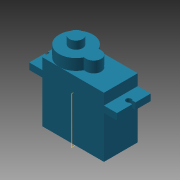
# Autodesk Inventor part: Servo
Saved by Autodesk Inventor 2014 SP1 (Build 180222100, 222)
## iProperties
Created: 2017-01-16
Part Number: Servo
Material: Generic
Document SubType Name: Modeling
Designer: danielsikar
Density: 1 g/cm^3
Appearance: Turquoise
Author: danielsikar
Autodesk Inventor part; units mm, degrees
ref_plane "YZ Plane" through (0, 0, 0) normal (1, 0, 0) x (0, 1, 0)
ref_plane "XZ Plane" through (0, 0, 0) normal (0, 1, 0) x (-1, 0, 0)
ref_plane "XY Plane" through (0, 0, 0) normal (0, 0, 1) x (1, 0, 0)
sketch "Sketch1" plane through (0, 0, 0) normal (0, 0, 1) x (1, 0, 0)
  line L0 (0, 0) -> (22.8, 0)
  line L1 (22.8, 0) -> (22.8, 12.5)
  line L2 (22.8, 12.5) -> (0, 12.5)
  line L3 (0, 12.5) -> (0, 0)
  dimension "d0" = 22.8
  dimension "d1" = 12.5
  constraints: 8 end point, 2 parallel, 1 horizontal, 1 perpendicular
  measures "d0" distance of L2.end L1.end
  measures "d1" distance of L1.end L0.end
extrude "Extrusion1" add sketch "Sketch1" along normal blind 22.1
sketch "Sketch2" plane through (22.8, 0, 0) normal (1, 0, 0) x (0, 0, -1)
  line L0 (0, 12.5) -> (-22.1, 12.5) projected
  line L1 (-22.1, 0) -> (-22.1, 12.5) projected
  line L2 (0, 0) -> (-22.1, 0) projected
  line L3 (-18, 12.5) -> (-15.6, 12.5)
  line L4 (-15.6, 12.5) -> (-15.6, 0)
  line L5 (-15.6, 0) -> (-18, 0)
  line L6 (-18, 0) -> (-18, 12.5)
  dimension "d4" = 2.4
  dimension "d5" = 4.1
  constraints: 8 end point, 2 parallel, 2 point on line, 1 horizontal, 1 perpendicular
  measures "d4" distance of L4.end L5.end
  measures "d5" distance between parallel lines of L6 L1
extrude "Extrusion2" add sketch "Sketch2" along normal blind 4.8 contours L4 L2 L6 L0
sketch "Sketch3" plane through (22.8, 0, 18) normal (0, 0, 1) x (1, 0, 0)
  line L0 (0, 0) -> (0, 12.5) projected
  circle A0 centre (2.9, 6.25) radius 1
  point P0 (-22.8, 0)
  dimension "d8" = 2
  dimension "d9" = 2.9
  constraints: 1 centre point
  measures "d8" diameter of A0
  measures "d9" distance from line of A0.centre L0
extrude "Extrusion3" cut sketch "Sketch3" against normal up to surface (2.4 mm away)
sketch "Sketch4" plane through (27.6, 0, 0) normal (1, 0, 0) x (0, 0, -1)
  line L0 (-18, 12.5) -> (-18, 0) projected
  line L1 (-15.6, 0) -> (-15.6, 12.5) projected
  line L2 (-18, 6.85) -> (-15.6, 6.85)
  line L3 (-15.6, 6.85) -> (-15.6, 5.65)
  line L4 (-15.6, 5.65) -> (-18, 5.65)
  line L5 (-18, 5.65) -> (-18, 6.85)
  point P0 (0, 0)
  point P1 (-15.6, 6.25)
  point P2 (-15.6, 6.25)
  dimension "d12" = 1.2
  constraints: 8 end point, 2 midpoint, 2 parallel, 2 point on line, 1 coincident, 1 horizontal, 1 perpendicular
  measures "d12" distance of L2.end L3.end
extrude "Extrusion4" cut sketch "Sketch4" against normal blind 2
ref_plane "Work Plane1" through (11.4, 0, 0) normal (1, 0, 0) x (0, 0, -1)
mirror "Mirror1" about plane through (11.4, 0, 0) normal (1, 0, 0) of "Extrusion2", "Extrusion3", "Extrusion4"
sketch "Sketch5" plane through (0, 0, 22.1) normal (0, 0, 1) x (1, 0, 0)
  line L0 (0, 0) -> (22.8, 0) projected
  line L1 (22.8, 0) -> (22.8, 12.5) projected
  line L2 (0, 12.5) -> (0, 0) projected
  arc A0 (11.8625, 9) -> (11.8625, 3.5) centre (6.25, 6.25) ccw
  arc A1 (12.8, 3.5) -> (12.8, 9) centre (12.8, 6.25) ccw
  line L3 (12.8, 9) -> (11.8625, 9)
  line L4 (12.8, 3.5) -> (11.8625, 3.5)
  point P0 (0, 6.25)
  dimension "d16" = 5.5
  dimension "d17" = 10
  constraints: 5 point on circle, 4 end point, 3 tangent, 2 centre point, 1 midpoint, 1 parallel, 1 perpendicular
  measures "d16" diameter of A1
  measures "d17" distance from line of L1 A1.centre
extrude "Extrusion5" add sketch "Sketch5" along normal blind 4.1 contours A0 L3 A1 L4
sketch "Sketch6" plane through (0, 0, 26.2) normal (0, 0, 1) x (1, 0, 0)
  arc A0 (11.8625, 9) -> (11.8625, 3.5) centre (6.25, 6.25) ccw projected
  circle A1 centre (6.25, 6.25) radius 2.45
  point P0 (0, 0)
  dimension "d20" = 4.9
  constraints: 1 centre point, 1 coincident
  measures "d20" diameter of A1
extrude "Extrusion6" add sketch "Sketch6" along normal blind 2.9
body "Solid1"
